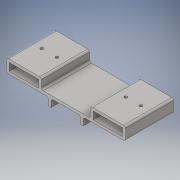
# Autodesk Inventor part: Up_Part_Robot
Saved by Autodesk Inventor 2016 (Build 200138000, 138)
## iProperties
Created: 2015-09-23
Part Number: Up_Part_Robot
Material: Generic
Document SubType Name: Modeling
Designer: fei
Density: 1 g/cm^3
Appearance: Default
Author: fei
Autodesk Inventor part; units mm, degrees
ref_plane "YZ Plane" through (0, 0, 0) normal (1, 0, 0) x (0, 1, 0)
ref_plane "XZ Plane" through (0, 0, 0) normal (0, 1, 0) x (-1, 0, 0)
ref_plane "XY Plane" through (0, 0, 0) normal (0, 0, 1) x (1, 0, 0)
sketch "Sketch1" plane through (0, 0, 0) normal (1, 0, 0) x (0, 1, 0)
  line L0 (38.1, 647.7) -> (-38.1, 647.7)
  line L1 (-38.1, 647.7) -> (-38.1, -647.7)
  line L2 (-38.1, -647.7) -> (38.1, -647.7)
  line L3 (38.1, -647.7) -> (38.1, 647.7)
  line L4 (0, 0) -> (486.9553, 0) construction
  point P0 (0, -647.7)
  dimension "d0" = 1295.4
  dimension "d1" = 76.2
  dimension "d2" = 647.7
  constraints: 10 end point, 2 horizontal, 2 parallel, 1 midpoint, 1 perpendicular, 1 vertical alignment
  measures "d0" distance of L2.end L0.start
  measures "d1" distance of L1.end L2.end
  measures "d2" distance of point (0, -647.7) L4.start
extrude "Extrusion1" add sketch "Sketch1" along normal blind 1600.2
sketch "Sketch2" plane through (0, 38.1, 647.7) normal (0, 1, 0) x (1, 0, 0)
  line L0 (1600.2, 0) -> (1600.2, 1295.4) projected
  line L1 (0, 0) -> (1600.2, 0) projected
  line L2 (1600.2, 1295.4) -> (1524, 1295.4)
  line L3 (1524, 1295.4) -> (1524, 0)
  line L4 (1524, 0) -> (1600.2, 0)
  line L5 (1600.2, 0) -> (1600.2, 1295.4)
  line L6 (1600.2, 1295.4) -> (1600.2, 0) projected
  point P0 (0, 647.7)
  dimension "d5" = 76.2
  constraints: 8 end point, 2 parallel, 1 horizontal, 1 perpendicular, 1 point on line
  measures "d5" distance of L4.end L3.end
extrude "Extrusion2" add sketch "Sketch2" along normal blind 279.4
sketch "Sketch3" plane through (1524, 38.1, -647.7) normal (-1, 0, 0) x (0, 0, 1)
  line L0 (0, -76.2) -> (0, 279.4) projected
  line L1 (1295.4, -76.2) -> (1295.4, 279.4) projected
  line L2 (0, 279.4) -> (1295.4, 279.4)
  line L3 (1295.4, 279.4) -> (1295.4, 203.2)
  line L4 (1295.4, 203.2) -> (0, 203.2)
  line L5 (0, 203.2) -> (0, 279.4)
  point P0 (647.7, -38.1)
  dimension "d8" = 76.2
  constraints: 8 end point, 2 parallel, 1 horizontal, 1 perpendicular, 1 point on line
  measures "d8" distance of L3.end L1.end
extrude "Extrusion3" add sketch "Sketch3" along normal blind 863.6
sketch "Sketch4" plane through (1524, 241.3, -647.7) normal (0, -1, 0) x (1, 0, 0)
  line L0 (-863.6, 1295.4) -> (-863.6, 0) projected
  line L1 (-1524, 0) -> (0, 0) projected
  line L2 (-863.6, 1295.4) -> (-787.4, 1295.4)
  line L3 (-787.4, 1295.4) -> (-787.4, 0)
  line L4 (-787.4, 0) -> (-863.6, 0)
  line L5 (-863.6, 0) -> (-863.6, 1295.4)
  point P0 (-1524, 647.7)
  dimension "d11" = 76.2
  constraints: 8 end point, 2 parallel, 1 horizontal, 1 perpendicular, 1 point on line
  measures "d11" distance of L3.end L4.end
extrude "Extrusion4" add sketch "Sketch4" along normal up to next
sketch "Sketch5" plane through (0, -38.1, -647.7) normal (0, -1, 0) x (1, 0, 0)
  line L0 (0, 1295.4) -> (1600.2, 1295.4) projected
  line L1 (0, 0) -> (1600.2, 0) projected
  line L2 (393.7, 1295.4) -> (469.9, 1295.4)
  line L3 (469.9, 1295.4) -> (469.9, 0)
  line L4 (469.9, 0) -> (393.7, 0)
  line L5 (393.7, 0) -> (393.7, 1295.4)
  point P0 (0, 647.7)
  dimension "d14" = 76.2
  dimension "d15" = 469.9
  constraints: 8 end point, 2 parallel, 2 point on line, 1 horizontal, 1 perpendicular
  measures "d14" distance of L2.end L2.start
  measures "d15" distance of L1.start L3.end
extrude "Extrusion5" add sketch "Sketch5" along normal blind 203.2
sketch "Sketch6" plane through (469.9, -38.1, 647.7) normal (1, 0, 0) x (0, 0, -1)
  point P0 (647.7, 38.1)
sketch "Sketch7" plane through (469.9, -38.1, 647.7) normal (1, 0, 0) x (0, 0, -1)
  circle A0 centre (323.85, -101.6) radius 38.1
  line L0 (0, 0) -> (0, -203.2) projected
  line L1 (1295.4, -203.2) -> (0, -203.2) projected
  point P0 (647.7, 38.1)
  dimension "d18" = 76.2
  dimension "d19" = 323.85
  dimension "d20" = 101.6
  constraints: 1 centre point
  measures "d18" diameter of A0
  measures "d19" distance from line of L0 A0.centre
  measures "d20" distance from line of L1 A0.centre
extrude "Extrusion6" cut sketch "Sketch7" against normal through all
pattern_linear "Rectangular Pattern1" count 3 spacing 317.5 along (0, 0, -1) of "Extrusion6"
fillet "Fillet1" radius 50.8 1 edges at (393.7, -38.1, 0)
sketch "Sketch8" plane through (0, 317.5, 647.7) normal (0, 1, 0) x (1, 0, 0)
  circle A0 centre (927.1, 685.8) radius 38.1
  line L0 (1600.2, 0) -> (660.4, 0) projected
  line L1 (660.4, 0) -> (660.4, 1295.4) projected
  circle A1 centre (1333.5, 685.8) radius 38.1
  point P0 (0, 647.7)
  dimension "d28" = 76.2
  dimension "d29" = 685.8
  dimension "d30" = 266.7
  dimension "d31" = 76.2
  dimension "d32" = 406.4
  constraints: 2 centre point, 1 horizontal alignment
  measures "d28" diameter of A0
  measures "d29" distance from line of L0 A0.centre
  measures "d30" distance from line of L1 A0.centre
  measures "d31" diameter of A1
  measures "d32" distance of A1.centre A0.centre
extrude "Extrusion7" cut sketch "Sketch8" along normal up to surface (76.2 mm away) from surface at -76.2
fillet "Fillet3" radius 50.8 4 edges at (1600.2, 317.5, 0) (660.4, 317.5, 0) (1600.2, -38.1, 0) (469.9, -38.1, 0)
mirror "Mirror1" about plane through (0, 0, 0) normal (1, 0, 0) of "Extrusion1", "Extrusion2", "Extrusion3", "Extrusion4", "Extrusion5", "Extrusion6", "Rectangular Pattern1", "Fillet1", "Extrusion7", "Fillet3"
body "Solid1"
